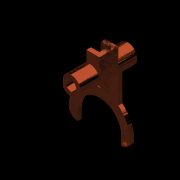
# Autodesk Inventor part: GearPawl
Saved by Autodesk Inventor 2022 (Build 260153000, 153)
## iProperties
Created: 2020-12-29
Part Number: GearPawl
Material: Generic
Document SubType Name: Modeling
Designer: jdski
Density: 1 g/cm^3
Appearance: Default
Author: jdski
Autodesk Inventor part; units mm, degrees
ref_plane "YZ Plane" through (0, 0, 0) normal (1, 0, 0) x (0, 1, 0)
ref_plane "XZ Plane" through (0, 0, 0) normal (0, 1, 0) x (-1, 0, 0)
ref_plane "XY Plane" through (0, 0, 0) normal (0, 0, 1) x (1, 0, 0)
sketch "Sketch1" plane through (0, 0, 0) normal (0, 0, 1) x (1, 0, 0)
  arc A0 (18.8242, 7.4512) -> (-10.2588, 7.4512) centre (4.2827, 7.4512) ccw
  arc A1 (24.8115, 5.3358) -> (-16.2461, 5.3358) centre (4.2827, 7.4512) ccw
  arc A2 (18.8242, 1.1012) -> (24.8115, 5.3358) centre (18.8242, 7.4512) ccw
  arc A3 (-16.2461, 5.3358) -> (-10.2588, 1.1012) centre (-10.2588, 7.4512) ccw
  line L0 (18.8242, 7.4512) -> (18.8242, 1.1012)
  line L1 (-10.2588, 7.4512) -> (-10.2588, 1.1012)
  circle A4 centre (10.6327, 44.7574) radius 3.429
  arc A5 (5.0765, 41.6832) -> (5.0765, 47.8316) centre (10.6327, 44.7574) ccw
  line L2 (5.0765, 28.0734) -> (5.0765, 47.8316)
  line L3 (16.9827, 44.7574) -> (16.9827, 23.7182)
  line L4 (16.9827, 44.7574) -> (16.9827, 58.2512)
  line L5 (16.9827, 58.2512) -> (8.2515, 58.2512)
  line L6 (8.2515, 58.2512) -> (8.2515, 50.644)
  line L7 (10.6327, 38.4074) -> (10.6327, 27.0875)
  line L8 (10.6327, 44.7574) -> (28.3027, 44.7574) construction
  point P0 (0, 0)
  dimension "d11" = 90
  constraints: 18 end point, 16 point on circle, 6 centre point, 1 horizontal, 1 point on line
  measures "d11" angle of L7 L8
extrude "Extrusion1" add sketch "Sketch1" against normal blind 2.667 contours A0 L1 A3 A1 A2 L0 | A1 L7 A5 L3 | L2 A5 L7 A1
extrude "Extrusion2" add sketch "Sketch1" against normal blind 12.7 contours A5 L2
extrude "Extrusion3" add sketch "Sketch1" along normal blind 25.4 contours A5 L2
extrude "Extrusion4" add sketch "Sketch1" along normal blind 12.7 contours A5 L6 L5 L4
sketch "Sketch2" plane through (8.2515, 58.2512, 0) normal (0, 1, 0) x (1, 0, 0)
  line L0 (8.7313, -12.7) -> (0, -12.7) projected
  line L1 (8.7313, 0) -> (8.7313, -12.7) projected
  line L2 (8.7313, 0) -> (0, 0) projected
  line L3 (0, -9.652) -> (5.6833, -9.652)
  line L4 (5.6833, -9.652) -> (5.6833, -3.048)
  line L5 (5.6833, -3.048) -> (0, -3.048)
  line L6 (0, -12.7) -> (0, -9.652)
  line L7 (0, -3.048) -> (0, 0)
  line L8 (0, 0) -> (0, -12.7) projected
  point P0 (-8.2515, 0)
  dimension "d8" = 3.048
  constraints: 10 end point, 1 collinear, 1 vertical, 2 other
  measures "d8" distance between parallel lines of L0 L3
extrude "Extrusion5" cut sketch "Sketch2" against normal up to surface contours L8 L5 L4 L3 round surface about axis through (10.6327, 44.7574, 0) along (0, 0, -1) radius 6.35 far side no
extrude "Extrusion6" add sketch "Sketch1" along normal blind 6.35 contours L2 A5 L7 A1
chamfer "Chamfer1" distance 9.525 distance2 6.35 1 edges at (7.8885, 27.7712, 6.35) measured on face at (7.9758, 28.2635, 6.35)
body "Solid1"
